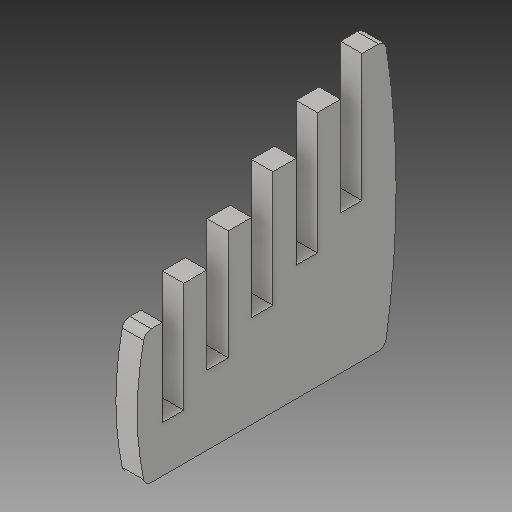
# Autodesk Inventor part: Head Frame
Saved by Autodesk Inventor 2019 (Build 230136000, 136)
## iProperties
Created: 2020-02-12
Part Number: Head Frame
Material: Generic
Document SubType Name: Modeling
Designer: student
Density: 1 g/cm^3
Appearance: Default
Author: student
Autodesk Inventor part; units mm, degrees
ref_plane "YZ Plane" through (0, 0, 0) normal (1, 0, 0) x (0, 1, 0)
ref_plane "XZ Plane" through (0, 0, 0) normal (0, 1, 0) x (-1, 0, 0)
ref_plane "XY Plane" through (0, 0, 0) normal (0, 0, 1) x (1, 0, 0)
sketch "Sketch1" plane through (0, 0, 0) normal (1, 0, 0) x (0, 1, 0)
  line L0 (0, 0) -> (58.42, 0) construction
  line L1 (58.42, 0) -> (58.42, -52.705) construction
  line L2 (58.42, -52.705) -> (0, -52.705) construction
  line L3 (0, -52.705) -> (0, 0) construction
  line L4 (0, 0) -> (0, -52.705)
  line L5 (0, -52.705) -> (58.42, -52.705) construction
  line L6 (29.21, -3.81) -> (10.16, -3.81)
  line L7 (10.16, -3.81) -> (10.16, -8.509)
  line L8 (10.16, -8.509) -> (34.29, -8.509)
  line L9 (34.29, -8.509) -> (34.29, -13.589)
  line L10 (34.29, -13.589) -> (15.24, -13.589)
  line L11 (15.24, -13.589) -> (15.24, -18.288)
  line L12 (29.21, -3.81) -> (29.21, 0)
  line L13 (0, 0) -> (29.21, 0) construction
  line L14 (15.24, -18.288) -> (39.37, -18.288)
  line L15 (39.37, -18.288) -> (39.37, -23.368)
  line L16 (39.37, -23.368) -> (20.32, -23.368)
  line L17 (20.32, -23.368) -> (20.32, -28.067)
  line L18 (20.32, -28.067) -> (45.72, -28.067)
  line L19 (45.72, -28.067) -> (45.72, -33.147)
  line L20 (58.42, -52.705) -> (58.42, -47.625)
  line L21 (58.42, -47.625) -> (30.48, -47.625)
  line L22 (30.48, -47.625) -> (30.48, -42.926)
  line L23 (30.48, -42.926) -> (52.07, -42.926)
  line L24 (52.07, -42.926) -> (52.07, -37.846)
  line L25 (52.07, -37.846) -> (25.4, -37.846)
  line L26 (25.4, -37.846) -> (25.4, -33.147)
  line L27 (25.4, -33.147) -> (45.72, -33.147)
  arc A0 (29.21, 0) -> (0, 0) centre (14.605, -61.7976) ccw
  arc A1 (0, -52.705) -> (58.42, -52.705) centre (29.21, 122.6792) ccw
  dimension "d0" = 52.705
  dimension "d1" = 58.42
  dimension "d2" = 4.699
  dimension "d3" = 3.81
  dimension "d5" = 5.08
  dimension "d6" = 5.08
  dimension "d7" = 4.699
  dimension "d8" = 10.16
  dimension "d9" = 19.05
  dimension "d10" = 19.05
  dimension "d11" = 5.08
  dimension "d12" = 4.699
  dimension "d13" = 5.08
  dimension "d14" = 19.05
  dimension "d15" = 5.08
  dimension "d18" = 4.699
  dimension "d19" = 4.699
  dimension "d22" = 5.08
  dimension "d28" = 5.08
  dimension "d35" = 63.5
  dimension "d36" = 177.8
  dimension "d39" = 5.08
  dimension "d40" = 6.35
  dimension "d42" = 5.08
  dimension "d43" = 6.35
  dimension "d44" = 6.35
  constraints: 56 end point, 14 perpendicular, 4 equal length, 4 point on circle, 4 vertical, 3 horizontal, 2 centre point, 1 midpoint, 1 point on line
  measures "d0" distance of L2.end L0.start
  measures "d1" distance of L1.end L2.end
  measures "d2" distance between parallel lines of L8 L6
  measures "d3" distance between parallel lines of L0 L6
  measures "d5" distance of L8.end L9.end
  measures "d6" distance from line of L10.end L7
  measures "d7" distance of L10.end L11.end
  measures "d8" distance between parallel lines of L3 L7
  measures "d9" distance of L6.start L6.end
  measures "d10" distance of L9.end L10.end
  measures "d11" distance of L14.end L15.end
  measures "d12" distance of L16.end L17.end
  measures "d13" distance between parallel lines of L11 L17
  measures "d14" distance of L15.end L16.end
  measures "d15" distance of L18.end L19.end
  measures "d18" distance of L25.end L26.end
  measures "d19" distance of L21.end L22.end
  measures "d22" distance of L23.end L24.end
  measures "d28" distance between parallel lines of L26 L22
  measures "d35" radius of A0
  measures "d36" radius of A1
  measures "d39" distance of L1.end L20.end
  measures "d40" distance between parallel lines of L20 L24
  measures "d42" distance between parallel lines of L17 L26
  measures "d43" distance between parallel lines of L15 L19
  measures "d44" distance between parallel lines of L19 L24
extrude "Extrusion1" add sketch "Sketch1" against normal blind 4.699
fillet "Fillet1" radius 1.7145 4 edges at (-2.3495, 29.21, 0) (-2.3495, 0, 0) (-2.3495, 0, -52.705) (-2.3495, 58.42, -52.705)
equation "\"d2\" = thick"
equation "\"d6\" = 0.5 * d8"
equation "\"d7\" = thick"
equation "\"d12\" = thick"
equation "\"d13\" = d6"
equation "\"d18\" = thick"
equation "\"d19\" = thick"
equation "\"thick\" = 4.699"
body "Solid1"
